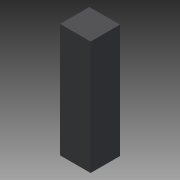
# Autodesk Inventor part: BPF
Saved by Autodesk Inventor 2014 (Build 180170000, 170)
## iProperties
Created: 2015-04-15
Part Number: BPF
Material: Generic
Document SubType Name: Modeling
Designer: Owner
Density: 1 g/cm^3
Appearance: Gray
Author: Owner
Autodesk Inventor part; units mm, degrees
ref_plane "YZ Plane" through (0, 0, 0) normal (1, 0, 0) x (0, 1, 0)
ref_plane "XZ Plane" through (0, 0, 0) normal (0, 1, 0) x (-1, 0, 0)
ref_plane "XY Plane" through (0, 0, 0) normal (0, 0, 1) x (1, 0, 0)
sketch "Sketch2" plane through (0, 0, 0) normal (0, 0, 1) x (1, 0, 0)
  line L0 (7.7849, -25.3234) -> (-1.4851, -25.3234)
  line L1 (-1.4851, -25.3234) -> (-1.4851, 9.2166)
  line L2 (-1.4851, 9.2166) -> (7.7849, 9.2166)
  line L3 (7.7849, 9.2166) -> (7.7849, -25.3234)
  point P0 (0, 0)
  dimension "d0" = 34.54
  dimension "d1" = 9.27
  constraints: 8 end point, 2 parallel, 1 horizontal, 1 perpendicular
  measures "d0" distance of L2.end L0.start
  measures "d1" distance of L1.end L2.end
extrude "Extrusion1" add sketch "Sketch2" along normal blind 8.89
body "Solid1"
